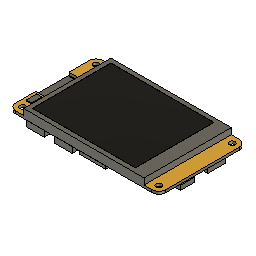
BusStop852 (Autodesk Fusion 360 archive; units mm, degrees)
design "Cheap Yellow Display"
part number: CYD
Autodesk Fusion 360 part; units mm, degrees
sketch "Sketch1" plane through (0, 0, 0) normal (0, 0, 1) x (1, 0, 0) in component "Display"
  line L0 (-39, 21) -> (39, 21) construction
  line L1 (39, 21) -> (39, -21) construction
  line L2 (39, -21) -> (-39, -21) construction
  line L3 (-39, -21) -> (-39, 21) construction
  line L4 (39, -25) -> (-39, -25)
  line L5 (-43, -21) -> (-43, 21)
  line L6 (-39, 25) -> (39, 25)
  line L7 (43, 21) -> (43, -21)
  arc A0 (43, 21) -> (39, 25) centre (39, 21) ccw
  arc A1 (39, -25) -> (43, -21) centre (39, -21) ccw
  arc A2 (-43, -21) -> (-39, -25) centre (-39, -21) ccw
  arc A3 (-39, 25) -> (-43, 21) centre (-39, 21) ccw
  circle A4 centre (-39, -21) radius 1.6
  circle A5 centre (39, -21) radius 1.6
  circle A6 centre (39, 21) radius 1.6
  circle A7 centre (-39, 21) radius 1.6
  dimension "d1" = 78
  dimension "d2" = 42
  dimension "d4" = 4
  dimension "d5" = 4
  dimension "d6" = 4
  dimension "d7" = 4
  dimension "d8" = 3.2
  dimension "d9" = 3.2
  dimension "d10" = 3.2
  dimension "d11" = 3.2
  constraint horizontal L0
  constraint vertical L1
  constraint horizontal L2
  constraint vertical L3
  constraint tangent L6 A0
  constraint tangent L7 A0
  constraint tangent L7 A1
  constraint tangent L4 A1
  constraint tangent L4 A2
  constraint tangent L5 A2
  constraint tangent L5 A3
  constraint tangent L6 A3
  constraint concentric A2 A4
  constraint concentric A1 A5
  constraint concentric A0 A6
  constraint concentric A3 A7
  measures "d1" distance of L0.start L0.end
  measures "d2" distance of L0.start L2.end
  measures "d4" radius of A0
  measures "d5" radius of A1
  measures "d6" radius of A2
  measures "d7" radius of A3
  measures "d8" diameter of A4
  measures "d9" diameter of A5
  measures "d10" diameter of A6
  measures "d11" diameter of A7
extrude "Extrude1" add sketch "Sketch1" along normal blind 1.5 in component "Display"
sketch "Sketch2" plane through (0, 0, 1.5) normal (0, 0, 1) x (-1, 0, 0) in component "Display"
  circle A0 centre (-39, 21) radius 1.6
  circle A1 centre (39, -21) radius 1.6
  circle A2 centre (39, 21) radius 1.6
  circle A3 centre (-39, -21) radius 1.6
  arc A4 (-43, -21) -> (-39, -25) centre (-39, -21) ccw
  line L0 (-39, -25) -> (39, -25)
  arc A5 (39, -25) -> (43, -21) centre (39, -21) ccw
  line L1 (43, -21) -> (43, 21)
  arc A6 (43, 21) -> (39, 25) centre (39, 21) ccw
  line L2 (39, 25) -> (-39, 25)
  arc A7 (-39, 25) -> (-43, 21) centre (-39, 21) ccw
  line L3 (-43, 21) -> (-43, -21)
  line L4 (34.5, -25) -> (-34.5, -25)
  line L5 (-34.5, -25) -> (-34.5, 25)
  line L6 (-34.5, 25) -> (34.5, 25)
  line L7 (34.5, 25) -> (34.5, -25)
  line L8 (41, 11) -> (38, 11)
  line L9 (38, 11) -> (38, 17)
  line L10 (38, 17) -> (41, 17)
  line L11 (41, 17) -> (41, 11)
  dimension "d14" = 69
  dimension "d15" = 50
  dimension "d16" = 8.5
  dimension "d19" = 6
  dimension "d20" = 2
  dimension "d21" = 8
  constraint horizontal L4
  constraint vertical L5
  constraint horizontal L6
  constraint vertical L7
  constraint horizontal L8
  constraint vertical L9
  constraint horizontal L10
  constraint vertical L11
  measures "d14" distance of L4.start L4.end
  measures "d15" distance of L4.start L6.end
  measures "d16" distance of L3 L5
  measures "d19" distance of L8.start L10.end
  measures "d20" distance of L1 L11
  measures "d21" distance of L2 L10
extrude "Extrude2" add sketch "Sketch2" along normal blind 3.5 contours L0 L2 L4 L5 L6 L7 in component "Display"
extrude "Extrude3" add sketch "Sketch2" along normal blind 0.5 contours L8 L9 L10 L11 in component "Display"
sketch "Sketch3" plane through (0, 0, 0) normal (0, 0, -1) x (1, 0, 0) in component "Display"
  circle A0 centre (39, 21) radius 1.6
  circle A1 centre (-39, -21) radius 1.6
  circle A2 centre (-39, 21) radius 1.6
  circle A3 centre (39, -21) radius 1.6
  arc A4 (39, -25) -> (43, -21) centre (39, -21) ccw
  line L0 (43, -21) -> (43, 21)
  arc A5 (43, 21) -> (39, 25) centre (39, 21) ccw
  line L1 (39, 25) -> (-39, 25)
  arc A6 (-39, 25) -> (-43, 21) centre (-39, 21) ccw
  line L2 (-43, 21) -> (-43, -21)
  arc A7 (-43, -21) -> (-39, -25) centre (-39, -21) ccw
  line L3 (-39, -25) -> (39, -25)
  line L4 (-17.6, -9) -> (-43, -9)
  line L5 (-43, -9) -> (-43, 9)
  line L6 (-43, 9) -> (-17.6, 9)
  line L7 (-17.6, 9) -> (-17.6, -9)
  line L8 (-10, 11.5) -> (-15, 11.5)
  line L9 (-15, 11.5) -> (-15, 16.5)
  line L10 (-15, 16.5) -> (-10, 16.5)
  line L11 (-10, 16.5) -> (-10, 11.5)
  line L12 (-31.9, -23.2) -> (-35.4, -23.2)
  line L13 (-35.4, -23.2) -> (-35.4, -17.2)
  line L14 (-35.4, -17.2) -> (-31.9, -17.2)
  line L15 (-31.9, -17.2) -> (-31.9, -23.2)
  line L16 (-31.4, -23.2) -> (-31.4, -17.2)
  line L17 (-31.4, -17.2) -> (-27.9, -17.2)
  line L18 (-27.9, -17.2) -> (-27.9, -23.2)
  line L19 (-27.9, -23.2) -> (-31.4, -23.2)
  line L20 (19, -23.8) -> (11.4, -23.8)
  line L21 (11.4, -23.8) -> (11.4, -20.6)
  line L22 (11.4, -20.6) -> (19, -20.6)
  line L23 (19, -20.6) -> (19, -23.8)
  line L24 (-36, -9) -> (-36, 9)
  line L25 (42, -14) -> (37.5, -14)
  line L26 (37.5, -14) -> (37.5, -4)
  line L27 (37.5, -4) -> (42, -4)
  line L28 (42, -4) -> (42, -14)
  line L29 (43.6, 5.4) -> (38.1, 5.4)
  line L30 (38.1, 5.4) -> (38.1, 13.2)
  line L31 (38.1, 13.2) -> (43.6, 13.2)
  line L32 (43.6, 13.2) -> (43.6, 5.4)
  line L33 (-22.8, 20.6) -> (-32.8, 20.6)
  line L34 (-32.8, 20.6) -> (-32.8, 24.9)
  line L35 (-32.8, 24.9) -> (-22.8, 24.9)
  line L36 (-22.8, 24.9) -> (-22.8, 20.6)
  line L37 (-16.8, 20.6) -> (-16.8, 24.9)
  line L38 (-16.8, 24.9) -> (-6.8, 24.9)
  line L39 (-6.8, 24.9) -> (-6.8, 20.6)
  line L40 (-6.8, 20.6) -> (-16.8, 20.6)
  line L41 (-2.6, 24.9) -> (12.4, 24.9)
  line L42 (12.4, 24.9) -> (12.4, 9.9)
  line L43 (12.4, 9.9) -> (-2.6, 9.9)
  line L44 (-2.6, 9.9) -> (-2.6, 24.9)
  dimension "d24" = 25.4
  dimension "d25" = 18
  dimension "d26" = 16
  dimension "d27" = 5
  dimension "d28" = 8.5
  dimension "d29" = 28
  dimension "d33" = 3.5
  dimension "d34" = 6
  dimension "d35" = 7.6
  dimension "d36" = 1.8
  dimension "d37" = 3.5
  dimension "d38" = 6
  dimension "d39" = 7.6
  dimension "d40" = 3.2
  dimension "d41" = 1.2
  dimension "d42" = 24
  dimension "d43" = 7
  dimension "d44" = 4.5
  dimension "d45" = 10
  dimension "d46" = 1
  dimension "d47" = 11
  dimension "d48" = 5.5
  dimension "d49" = 7.8
  dimension "d50" = 0.6
  dimension "d51" = 11.8
  dimension "d52" = 10
  dimension "d53" = 4.3
  dimension "d54" = 10.2
  dimension "d55" = 10
  dimension "d56" = 4.3
  dimension "d92" = 0.1
  dimension "d93" = 40.4
  constraint horizontal L4
  constraint vertical L5
  constraint horizontal L6
  constraint vertical L7
  constraint horizontal L8
  constraint vertical L9
  constraint horizontal L10
  constraint vertical L11
  constraint horizontal L12
  constraint vertical L13
  constraint horizontal L14
  constraint vertical L15
  constraint horizontal L19
  constraint vertical L16
  constraint horizontal L17
  constraint vertical L18
  constraint horizontal L20
  constraint vertical L21
  constraint horizontal L22
  constraint vertical L23
  constraint coincident L4 L24.start
  constraint coincident L6 L24.end
  constraint perpendicular L6 L24
  constraint horizontal L25
  constraint vertical L26
  constraint horizontal L27
  constraint vertical L28
  constraint horizontal L29
  constraint vertical L30
  constraint horizontal L31
  constraint vertical L32
  constraint horizontal L33
  constraint vertical L34
  constraint horizontal L35
  constraint vertical L36
  constraint horizontal L40
  constraint vertical L37
  constraint horizontal L38
  constraint vertical L39
  constraint horizontal L41
  constraint vertical L42
  constraint horizontal L43
  constraint vertical L44
  measures "d24" distance of L4.start L4.end
  measures "d25" distance of L4.start L6.end
  measures "d26" distance of L1 L6
  measures "d27" distance of L8.start L8.end
  measures "d28" distance of L1 L9.end
  measures "d29" distance of L2 L9.end
  measures "d33" distance of L12.start L12.end
  measures "d34" distance of L12.start L14.end
  measures "d35" horizontal distance of L2.end L12.end
  measures "d36" vertical distance of A7.end L12.end
  measures "d37" distance of L16.start L18.end
  measures "d38" distance of L18.end L17.end
  measures "d39" distance of L20.start L20.end
  measures "d40" distance of L20.start L22.end
  measures "d41" distance of L3 L20.end
  measures "d42" distance of A4.end L23
  measures "d43" distance of L5 L24
  measures "d44" distance of L25.start L25.end
  measures "d45" distance of L25.start L27.end
  measures "d46" distance of L0 L28
  measures "d47" distance of L3 L25
  measures "d48" distance of L29.start L29.end
  measures "d49" distance of L29.start L31.end
  measures "d50" distance of L0 L32
  measures "d51" distance of L1 L31
  measures "d52" distance of L33.start L33.end
  measures "d53" distance of L33.start L35.end
  measures "d54" distance of A6.end L34
  measures "d55" distance of L39.end L37.start
  measures "d56" distance of L38.end L39.end
  measures "d92" distance of L1 L41
  measures "d93" distance of L2 L44
extrude "Extrude4" add sketch "Sketch3" along normal blind 3 contours L4 L6 L7 L24 in component "Display"
extrude "Extrude5" add sketch "Sketch3" along normal blind 1 contours L2 L4 L5 L6 L24 in component "Display"
extrude "Extrude6" add sketch "Sketch3" along normal blind 3.5 contours L25 L26 L27 L28 | L33 L34 L35 L36 | L37 L38 L39 L40 in component "Display"
extrude "Extrude7" add sketch "Sketch3" along normal blind 1.5 contours L8 L9 L10 L11 in component "Display"
extrude "Extrude8" add sketch "Sketch3" along normal blind 2.5 contours L0 L29 L30 L31 | L0 L29 L31 L32 in component "Display"
extrude "Extrude9" add sketch "Sketch3" along normal blind 1.8 contours L41 L42 L43 L44 in component "Display"
extrude "Extrude10" add sketch "Sketch3" along normal blind 4.6 contours L20 L21 L22 L23 in component "Display"
extrude "Extrude11" add sketch "Sketch3" along normal blind 3.7 contours L12 L13 L14 L15 | L16 L17 L18 L19 in component "Display"
sketch "Sketch4" plane through (0, 0, -3.7) normal (0, 0, -1) x (1, 0, 0) in component "Display"
  line L0 (-27.9, -23.2) -> (-27.9, -17.2)
  line L1 (-27.9, -17.2) -> (-31.4, -17.2)
  line L2 (-31.4, -17.2) -> (-31.4, -23.2)
  line L3 (-31.4, -23.2) -> (-27.9, -23.2)
  line L4 (-28.9, -21.7) -> (-30.4, -21.7)
  line L5 (-30.4, -21.7) -> (-30.4, -18.7)
  line L6 (-30.4, -18.7) -> (-28.9, -18.7)
  line L7 (-28.9, -18.7) -> (-28.9, -21.7)
  line L8 (-29.65, -23.2) -> (-29.65, -24) construction
  line L9 (-31.4, -20.2) -> (-32, -20.2) construction
  line L10 (-35.4, -17.2) -> (-31.9, -17.2)
  line L11 (-31.9, -17.2) -> (-31.9, -23.2)
  line L12 (-35.4, -23.2) -> (-35.4, -17.2)
  line L13 (-31.9, -23.2) -> (-35.4, -23.2)
  line L14 (-33.65, -23.2) -> (-33.65, -24) construction
  line L15 (-35.4, -20.2) -> (-36, -20.2) construction
  line L16 (-34.4, -18.7) -> (-32.9, -18.7)
  line L17 (-32.9, -18.7) -> (-32.9, -21.7)
  line L18 (-32.9, -21.7) -> (-34.4, -21.7)
  line L19 (-34.4, -21.7) -> (-34.4, -18.7)
  dimension "d73" = 1.5
  dimension "d74" = 3
  dimension "d75" = 1.5
  dimension "d76" = 3
  constraint horizontal L4
  constraint vertical L5
  constraint horizontal L6
  constraint vertical L7
  constraint midpoint L3 L8.start
  constraint perpendicular L3 L8
  constraint midpoint L2 L9.start
  constraint perpendicular L2 L9
  constraint symmetric L5 L7 L8
  constraint symmetric L4 L6 L9
  constraint midpoint L13 L14.start
  constraint perpendicular L13 L14
  constraint midpoint L12 L15.start
  constraint perpendicular L12 L15
  constraint horizontal L18
  constraint vertical L19
  constraint horizontal L16
  constraint vertical L17
  constraint symmetric L15 L16 L18
  constraint symmetric L14 L17 L19
  measures "d73" distance of L4.start L4.end
  measures "d74" distance of L4.start L6.end
  measures "d75" distance of L17.end L18.end
  measures "d76" distance of L17.end L16.end
extrude "Extrude12" add sketch "Sketch4" along normal blind 1 contours L4 L5 L6 L7 | L16 L17 L18 L19 in component "Display"
sketch "Sketch5" plane through (0, 0, -1.5) normal (0, 0, -1) x (1, 0, 0) in component "Display"
  line L0 (-10, 16.5) -> (-15, 16.5)
  line L1 (-15, 16.5) -> (-15, 11.5)
  line L2 (-15, 11.5) -> (-10, 11.5)
  line L3 (-10, 11.5) -> (-10, 16.5)
  line L4 (-15, 16.5) -> (-10, 16.5)
  line L5 (-10, 16.5) -> (-10, 11.5)
  line L6 (-15, 11.5) -> (-15, 16.5)
  line L7 (-10, 11.5) -> (-15, 11.5)
  line L8 (-15, 16.5) -> (-10, 11.5) construction
  circle A0 centre (-12.5, 14) radius 2
  dimension "d79" = 4
  constraint coincident L0.end L1.start
  constraint coincident L2.end L3.start
  constraint midpoint L8 A0.centre
  measures "d79" diameter of A0
extrude "Extrude13" add sketch "Sketch5" along normal blind 0.1 contours A0 in component "Display"
sketch "Sketch6" plane through (0, 0, 5) normal (0, 0, 1) x (-1, 0, 0) in component "Display"
  line L0 (34.5, 25) -> (-34.5, 25)
  line L1 (-34.5, 25) -> (-34.5, -25)
  line L2 (-34.5, -25) -> (34.5, -25)
  line L3 (34.5, -25) -> (34.5, 25)
  line L4 (32, -22.5) -> (-27, -22.5)
  line L5 (-27, -22.5) -> (-27, 22.5)
  line L6 (-27, 22.5) -> (32, 22.5)
  line L7 (32, 22.5) -> (32, -22.5)
  line L8 (34.5, 0) -> (42, 0) construction
  line L9 (43, -21) -> (43, 21)
  line L10 (43, -9.5) -> (36.8, -9.5)
  line L11 (36.8, -9.5) -> (36.8, 9.5)
  line L12 (36.8, 9.5) -> (43, 9.5)
  line L13 (43, 9.5) -> (43, -9.5)
  dimension "d82" = 59
  dimension "d83" = 45
  dimension "d84" = 2.5
  dimension "d85" = 6.2
  dimension "d86" = 19
  constraint horizontal L4
  constraint vertical L5
  constraint horizontal L6
  constraint vertical L7
  constraint midpoint L3 L8.start
  constraint perpendicular L3 L8
  constraint symmetric L4 L6 L8
  constraint horizontal L10
  constraint vertical L11
  constraint horizontal L12
  constraint vertical L13
  constraint coincident L9 L10.start
  constraint symmetric L8 L10 L12
  measures "d82" distance of L4.start L4.end
  measures "d83" distance of L4.start L6.end
  measures "d84" distance of L3 L7
  measures "d85" distance of L10.start L10.end
  measures "d86" distance of L10.start L12.end
extrude "Extrude14" add sketch "Sketch6" along normal blind 0.1 contours L4 L5 L6 L7 in component "Display"
extrude "Extrude15" cut sketch "Sketch6" against normal up to surface (1.5 mm away) from surface at -3.5 contours L9 L10 L11 L12 L13 in component "Display"
component "Display" placed x (1, 0, 0) y (0, 1, 0) z (0, 0, 1) at (0, 0, 0)
equation "BORDER_W = 18.5 mm"
equation "SHELL = 1.8 mm"
equation "BORDER_H = 5 mm"
equation "TOLERANCE = 0.1 mm"
equation "CHAMFER = 0.6 mm"
equation "DEPTH = 15 mm"
equation "CATCH_WIDTH = 75 mm"
equation "LEG_WIDTH = 10 mm"

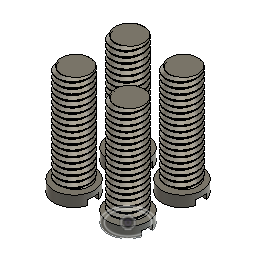
design "Screws"
Autodesk Fusion 360 part; units mm, degrees
sketch "Sketch1" plane through (0, 0, 0) normal (0, 1, 0) x (1, 0, 0)
  circle A0 centre (0, 0) radius 1.55
  circle A1 centre (0, 0) radius 1.85
  dimension "d1" = 3.1
  dimension "d4" = 3.7
  constraint coincident A0.centre A1.centre
  measures "d1" diameter of A0
  measures "d4" diameter of A1
extrude "Extrude1" add sketch "Sketch1" along normal blind 10 contours A0 makes body 1
extrude "Extrude2" add sketch "Sketch1" along normal blind 1 bodies 1
thread "Thread1" "ISO Metric profile 3.0 M3x0.5 M3x0.5 6g" major diameter 2.927 minor diameter 2.3555 pitch 0.5 angle 60 modelled right hand crest width 0.0713 on face at (1.5423, 4, 0.1543) crest through (1.4635, 0.875, 0) on bodies 1
sketch "Sketch2" plane through (0, 0, 0) normal (0, 1, 0) x (1, 0, 0)
  line L0 (1.8832, 0.5) -> (-1.8832, 0.5)
  line L1 (-1.8832, 0.5) -> (-1.8832, -0.5)
  line L2 (-1.8832, -0.5) -> (1.8832, -0.5)
  line L3 (1.8832, -0.5) -> (1.8832, 0.5)
  line L4 (1.8832, 0.5) -> (-1.8832, -0.5) construction
  line L5 (-1.8832, 0.5) -> (1.8832, -0.5) construction
  dimension "d9" = 1
  constraint horizontal L0
  constraint perpendicular L0 L1
  constraint parallel L0 L2
  constraint parallel L1 L3
  constraint coincident L4 origin
  constraint coincident L5 origin
  measures "d9" distance of L0.end L1.end
extrude "Extrude3" cut sketch "Sketch2" along normal blind 0.5 bodies 1
copy_body "CopyPasteBodies1" bodies 1 makes body 2
move_body "Move1" bodies 2 to x (1, 0, 0) y (0, 1, 0) z (0, 0, 1) at (0, 0, -5)
copy_body "CopyPasteBodies2" bodies 1 2 makes body 3 makes body 4
move_body "Move2" bodies 3 4 to x (1, 0, 0) y (0, 1, 0) z (0, 0, 1) at (-5, 0, 0)
